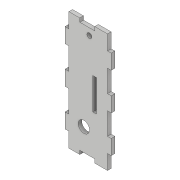
# Autodesk Inventor part: costat1
Saved by Autodesk Inventor 2019 (Build 230136000, 136)
## iProperties
Created: 2018-09-21
Part Number: costat1
Material: Genérico
Document SubType Name: Modeling
Designer: lmacia
Density: 1 g/cm^3
Appearance: Valor por defecto
Author: lmacia
Autodesk Inventor part; units mm, degrees
ref_plane "YZ Plane" through (0, 0, 0) normal (1, 0, 0) x (0, 1, 0)
ref_plane "XZ Plane" through (0, 0, 0) normal (0, 1, 0) x (-1, 0, 0)
ref_plane "XY Plane" through (0, 0, 0) normal (0, 0, 1) x (1, 0, 0)
sketch "Boceto1" plane through (0, 0, 0) normal (0, 0, 1) x (-1, 0, 0)
  line L0 (-18.892, -36.3978) -> (-15.842, -36.3978)
  line L1 (-15.842, -36.3978) -> (-15.842, -48.4963)
  line L2 (-15.842, -48.4963) -> (-5.3194, -48.4963)
  line L3 (-5.3194, -48.4963) -> (-5.3194, -45.4463)
  line L4 (-5.3194, -45.4463) -> (6.8808, -45.4463)
  line L5 (6.8808, -45.4463) -> (6.8808, -48.4963)
  line L6 (6.8808, -48.4963) -> (9.213, -48.4963)
  line L7 (9.213, -48.4963) -> (15.8784, -48.4963)
  line L8 (15.8784, -48.4963) -> (15.8784, -47.9533)
  line L9 (15.8784, -47.9533) -> (15.8784, -45.4463)
  line L10 (15.8784, -45.4463) -> (15.8784, -36.3641)
  line L11 (15.8784, -36.3641) -> (18.9284, -36.3641)
  line L12 (18.9284, -36.3641) -> (18.9284, -24.1977)
  line L13 (18.9288, -24.1977) -> (15.8806, -24.1977)
  line L14 (15.8761, -24.2652) -> (15.8784, -24.1977)
  line L15 (15.8806, -24.1977) -> (15.8797, -10.139)
  line L16 (15.8797, -10.139) -> (15.8784, -6.1009)
  line L17 (15.8761, -6.1684) -> (15.8784, -6.1009)
  line L18 (15.8784, -6.1009) -> (18.9284, -6.1009)
  line L19 (18.9284, -6.1009) -> (18.9284, 6.0992)
  line L20 (18.9284, 6.0992) -> (15.8784, 6.0992)
  line L21 (15.8784, 6.0992) -> (15.8784, 24.1961)
  line L22 (15.8784, 24.1961) -> (18.9284, 24.1961)
  line L23 (18.9284, 24.1961) -> (18.9284, 36.3962)
  line L24 (18.9284, 36.3962) -> (15.8784, 36.3962)
  line L25 (15.8784, 36.3962) -> (15.8784, 45.4446)
  line L26 (15.8784, 45.4446) -> (15.8784, 48.4947)
  line L27 (15.8784, 48.4947) -> (6.8808, 48.4947)
  line L28 (6.8808, 48.4947) -> (6.8808, 45.4446)
  line L29 (6.8808, 45.4446) -> (-3.6418, 45.4446)
  line L30 (-3.6418, 45.4446) -> (-5.3194, 45.4446)
  line L31 (-5.3194, 45.4446) -> (-5.3194, 48.4947)
  line L32 (-5.3194, 48.4947) -> (-15.842, 48.4947)
  line L33 (-15.842, 48.4947) -> (-15.842, 36.3962)
  line L34 (-15.842, 36.3962) -> (-18.892, 36.3962)
  line L35 (-18.892, 36.3962) -> (-18.892, 24.1961)
  line L36 (-18.892, 24.1961) -> (-15.842, 24.1961)
  line L37 (-15.842, 24.1961) -> (-15.842, 6.0992)
  line L38 (-15.842, 6.0992) -> (-18.892, 6.0992)
  line L39 (-18.892, 6.0992) -> (-18.892, -6.1009)
  line L40 (-18.892, -6.1009) -> (-15.842, -6.1009)
  line L41 (-15.842, -6.1009) -> (-15.842, -24.1977)
  line L42 (-15.842, -24.1977) -> (-17.8753, -24.1977)
  line L43 (-17.8753, -24.1977) -> (-18.892, -24.1977)
  line L44 (-18.892, -24.1977) -> (-18.892, -36.3978)
  line L45 (-6.6919, -12.9634) -> (-6.6919, 12.8601)
  line L46 (-6.6919, 12.8601) -> (-3.8452, 12.8601)
  line L47 (-3.8452, 12.8601) -> (-3.8452, -12.9634)
  line L48 (-3.8452, -12.9634) -> (-6.6919, -12.9634)
  circle A0 centre (3.5759, 27.1591) radius 4.6767
  circle A1 centre (-0.9985, -39.8545) radius 2.0334
  point P0 (0, 0)
  dimension "d2" = 37.8204
  dimension "d3" = 96.991
  constraints: 98 end point, 2 centre point, 1 horizontal, 1 point on line
  measures "d2" distance between parallel lines of L44 L12
  measures "d3" distance between parallel lines of L32 L2
extrude "Extrusión1" add sketch "Boceto1" along normal blind 3
